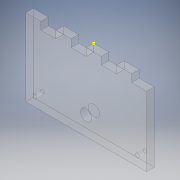
# Autodesk Inventor part: structural
Saved by Autodesk Inventor 2018 (Build 220112000, 112)
## iProperties
Created: 2018-10-03
Part Number: structural
Material: Polycarbonate, Clear
Document SubType Name: Modeling
Designer: Jayden
Density: 1.2 g/cm^3
Appearance: Polycarbonate - Clear
Author: Jayden
Autodesk Inventor part; units mm, degrees
ref_plane "YZ Plane" through (0, 0, 0) normal (1, 0, 0) x (0, 1, 0)
ref_plane "XZ Plane" through (0, 0, 0) normal (0, 1, 0) x (-1, 0, 0)
ref_plane "XY Plane" through (0, 0, 0) normal (0, 0, 1) x (1, 0, 0)
sketch "Sketch1" plane through (0, 0, 0) normal (0, 0, 1) x (1, 0, 0)
  circle A0 centre (0, 7.8) radius 4.7625
  circle A1 centre (-43, 0) radius 1.5875
  circle A2 centre (43, 0) radius 1.5875
  line L0 (-50.8, 56.695) -> (-38.1, 56.695)
  line L1 (50.8, -8.075) -> (-50.8, -8.075)
  line L2 (-50.8, -8.075) -> (-50.8, 56.695)
  line L3 (-50.8, 56.695) -> (-38.1, 56.695)
  line L4 (-38.1, 56.695) -> (-38.1, 50.345)
  line L5 (-50.8, 50.345) -> (-50.8, 56.695)
  line L6 (-38.1, 50.345) -> (-25.4, 50.345)
  line L7 (-25.4, 50.345) -> (-25.4, 56.695)
  line L8 (-38.1, 56.695) -> (-38.1, 50.345)
  line L9 (-12.7, 50.345) -> (-12.7, 56.695)
  line L10 (-12.7, 56.695) -> (-25.4, 56.695)
  line L11 (-25.4, 56.695) -> (-25.4, 50.345)
  line L12 (0, 56.695) -> (0, 50.345)
  line L13 (0, 50.345) -> (-12.7, 50.345)
  line L14 (-12.7, 50.345) -> (-12.7, 56.695)
  line L15 (12.7, 50.345) -> (12.7, 56.695)
  line L16 (12.7, 56.695) -> (0, 56.695)
  line L17 (0, 56.695) -> (0, 50.345)
  line L18 (25.4, 56.695) -> (25.4, 50.345)
  line L19 (25.4, 50.345) -> (12.7, 50.345)
  line L20 (12.7, 50.345) -> (12.7, 56.695)
  line L21 (25.4, 56.695) -> (38.1, 56.695)
  line L22 (38.1, 56.695) -> (38.1, 50.345)
  line L23 (25.4, 50.345) -> (25.4, 56.695)
  line L24 (38.1, 50.345) -> (50.8, 50.345)
  line L25 (38.1, 56.695) -> (38.1, 50.345)
  line L26 (0, 56.695) -> (12.7, 56.695)
  line L27 (25.4, 56.695) -> (38.1, 56.695)
  line L28 (50.8, 50.345) -> (50.8, -8.075)
  point P0 (0, 0)
  dimension "d0" = 9.525
  dimension "d1" = 3.175
  dimension "d2" = 3.175
  dimension "d6" = 0
  dimension "d7" = 101.6
  dimension "d13" = 43
  dimension "d14" = 43
  dimension "d16" = 15.875
  dimension "d17" = 7.8
  dimension "d18" = 7.8
  dimension "d19" = 48.895
  dimension "d21" = 12.7
  dimension "d22" = 6.35
  dimension "d23" = 12.7
  dimension "d24" = 12.7
  dimension "d25" = 6.35
  dimension "d26" = 6.35
  dimension "d27" = 12.7
  dimension "d28" = 6.35
  dimension "d29" = 12.7
  dimension "d30" = 6.35
  dimension "d31" = 12.7
  dimension "d32" = 6.35
  constraints: 58 end point, 11 parallel, 7 horizontal, 6 perpendicular, 3 centre point, 1 point on line
  measures "d0" diameter of A0
  measures "d1" diameter of A1
  measures "d2" diameter of A2
  measures "d6" vertical distance of point (0, 0) A1.centre
  measures "d7" distance of L1.start L1.end
  measures "d13" distance of point (0, 0) A1.centre
  measures "d14" distance of A2.centre point (0, 0)
  measures "d16" distance from line of L1 A0.centre
  measures "d17" vertical distance of A1.centre A0.centre
  measures "d18" vertical distance of A2.centre A0.centre
  measures "d19" distance from line of L0 A0.centre
  measures "d21" distance of L4.end L5.start
  measures "d22" distance of L3.end L4.end
  measures "d23" distance of L0.end L7.end
  measures "d24" distance of L10.end L9.end
  measures "d25" distance of L9.end L9.start
  measures "d26" distance of L12.start L12.end
  measures "d27" distance of L16.end L15.end
  measures "d28" distance of L15.end L15.start
  measures "d29" distance of L18.end L19.end
  measures "d30" distance of L18.start L18.end
  measures "d31" distance of L22.end L23.start
  measures "d32" distance of L21.end L22.end
extrude "Extrusion1" add sketch "Sketch1" along normal blind 6.35
sketch "Sketch2" plane through (-50.8, 56.695, 0) normal (0, 1, 0) x (1, 0, 0)
  point P0 (50.8, 0)
body "Solid1"
